Autodesk Fusion 360 part; units mm, degrees
(part 4 of 4)
  spline S181 degree 3 poles (233.08, 32.65) (233.08, 32.7604) (232.9906, 32.85) (232.88, 32.85) knots 6 6 6 6 7 7 7 7
  line L275 (233.08, 32.65) -> (233.08, 19.05)
  spline S182 degree 3 poles (232.88, 18.85) (232.9906, 18.85) (233.08, 18.9395) (233.08, 19.05) knots 4 4 4 4 5 5 5 5
  line L276 (232.88, 18.85) -> (219.2802, 18.85)
  spline S183 degree 3 poles (219.08, 19.05) (219.08, 18.9395) (219.1696, 18.85) (219.2802, 18.85) knots 2 2 2 2 3 3 3 3
  line L277 (219.08, 19.05) -> (219.08, 32.65)
  spline S184 degree 3 poles (219.2802, 32.85) (219.1696, 32.85) (219.08, 32.7604) (219.08, 32.65) knots 0 0 0 0 1 1 1 1
  line L278 (219.2802, 32.85) -> (232.88, 32.85)
  spline S185 degree 3 poles (224.0301, 51.9) (223.9197, 51.9) (223.8301, 51.8104) (223.8301, 51.7) knots 6 6 6 6 7 7 7 7
  line L279 (224.0301, 51.9) -> (237.6301, 51.9)
  spline S186 degree 3 poles (237.8301, 51.7) (237.8301, 51.8104) (237.7405, 51.9) (237.6301, 51.9) knots 4 4 4 4 5 5 5 5
  line L280 (237.8301, 51.7) -> (237.8301, 38.1)
  spline S187 degree 3 poles (237.6301, 37.9) (237.7405, 37.9) (237.8301, 37.9895) (237.8301, 38.1) knots 2 2 2 2 3 3 3 3
  line L281 (237.6301, 37.9) -> (224.0301, 37.9)
  spline S188 degree 3 poles (223.8301, 38.1) (223.8301, 37.9895) (223.9197, 37.9) (224.0301, 37.9) knots 0 0 0 0 1 1 1 1
  line L282 (223.8301, 38.1) -> (223.8301, 51.7)
  line L283 (248.0298, 7.33) -> (248.8547, 7.33)
  line L284 (248.8547, 7.33) -> (248.8547, 13.53)
  line L285 (248.8547, 13.53) -> (250.6798, 13.53)
  line L286 (250.6798, 13.53) -> (250.6798, 14.78)
  line L287 (250.6798, 14.78) -> (253.6798, 14.78)
  line L288 (253.6798, 14.78) -> (253.6798, 13.53)
  line L289 (253.6798, 13.53) -> (255.5046, 13.53)
  line L290 (255.5046, 13.53) -> (255.5046, 11.03)
  line L291 (255.5046, 11.03) -> (257.18, 11.03)
  line L292 (257.18, 11.03) -> (257.18, 13.6)
  spline S189 degree 3 poles (257.3802, 13.8) (257.2696, 13.8) (257.18, 13.7104) (257.18, 13.6) knots 28 28 28 28 29 29 29 29
  line L293 (257.3802, 13.8) -> (270.98, 13.8)
  spline S190 degree 3 poles (271.18, 13.6) (271.18, 13.7104) (271.0906, 13.8) (270.98, 13.8) knots 26 26 26 26 27 27 27 27
  line L294 (271.18, 13.6) -> (271.18, 11.03)
  line L295 (271.18, 11.03) -> (272.8557, 11.03)
  line L296 (272.8557, 11.03) -> (272.8557, 13.53)
  line L297 (272.8557, 13.53) -> (274.6807, 13.53)
  line L298 (274.6807, 13.53) -> (274.6807, 14.78)
  line L299 (274.6807, 14.78) -> (277.6807, 14.78)
  line L300 (277.6807, 14.78) -> (277.6807, 13.53)
  line L301 (277.6807, 13.53) -> (279.5058, 13.53)
  line L302 (279.5058, 13.53) -> (279.5058, 7.33)
  line L303 (279.5058, 7.33) -> (280.3307, 7.33)
  line L304 (280.3307, 7.33) -> (280.3307, 4.32)
  line L305 (280.3307, 4.32) -> (279.5058, 4.32)
  line L306 (279.5058, 4.32) -> (279.5058, 1.32)
  line L307 (279.5058, 1.32) -> (272.8557, 1.32)
  line L308 (272.8557, 1.32) -> (272.8557, 3.82)
  line L309 (272.8557, 3.82) -> (271.18, 3.82)
  line L310 (271.18, 3.82) -> (271.18, 0)
  spline S191 degree 3 poles (270.98, -0.2) (271.0906, -0.2) (271.18, -0.1105) (271.18, 0) knots 8 8 8 8 9 9 9 9
  line L311 (270.98, -0.2) -> (257.3802, -0.2)
  spline S192 degree 3 poles (257.18, 0) (257.18, -0.1105) (257.2696, -0.2) (257.3802, -0.2) knots 6 6 6 6 7 7 7 7
  line L312 (257.18, 0) -> (257.18, 3.82)
  line L313 (257.18, 3.82) -> (255.5046, 3.82)
  line L314 (255.5046, 3.82) -> (255.5046, 1.32)
  line L315 (255.5046, 1.32) -> (248.8547, 1.32)
  line L316 (248.8547, 1.32) -> (248.8547, 4.32)
  line L317 (248.8547, 4.32) -> (248.0298, 4.32)
  line L318 (248.0298, 4.32) -> (248.0298, 7.33)
  spline S193 degree 3 poles (280.5, 56.95) (280.6104, 56.95) (280.7, 57.0395) (280.7, 57.15) knots 6 6 6 6 7 7 7 7
  line L319 (280.5, 56.95) -> (266.9, 56.95)
  spline S194 degree 3 poles (266.7, 57.15) (266.7, 57.0395) (266.7896, 56.95) (266.9, 56.95) knots 4 4 4 4 5 5 5 5
  line L320 (266.7, 57.15) -> (266.7, 70.75)
  spline S195 degree 3 poles (266.9, 70.95) (266.7896, 70.95) (266.7, 70.8604) (266.7, 70.75) knots 2 2 2 2 3 3 3 3
  line L321 (266.9, 70.95) -> (280.5, 70.95)
  spline S196 degree 3 poles (280.7, 70.75) (280.7, 70.8604) (280.6104, 70.95) (280.5, 70.95) knots 0 0 0 0 1 1 1 1
  line L322 (280.7, 70.75) -> (280.7, 57.15)
  spline S197 degree 3 poles (299.55, -0.2) (299.6604, -0.2) (299.75, -0.1105) (299.75, 0) knots 6 6 6 6 7 7 7 7
  line L323 (299.55, -0.2) -> (285.95, -0.2)
  spline S198 degree 3 poles (285.75, 0) (285.75, -0.1105) (285.8396, -0.2) (285.95, -0.2) knots 4 4 4 4 5 5 5 5
  line L324 (285.75, 0) -> (285.75, 13.6)
  spline S199 degree 3 poles (285.95, 13.8) (285.8396, 13.8) (285.75, 13.7104) (285.75, 13.6) knots 2 2 2 2 3 3 3 3
  line L325 (285.95, 13.8) -> (299.55, 13.8)
  spline S200 degree 3 poles (299.75, 13.6) (299.75, 13.7104) (299.6604, 13.8) (299.55, 13.8) knots 0 0 0 0 1 1 1 1
  line L326 (299.75, 13.6) -> (299.75, 0)
  spline S201 degree 3 poles (280.5, 76) (280.6104, 76) (280.7, 76.0895) (280.7, 76.2) knots 6 6 6 6 7 7 7 7
  line L327 (280.5, 76) -> (266.9, 76)
  spline S202 degree 3 poles (266.7, 76.2) (266.7, 76.0895) (266.7896, 76) (266.9, 76) knots 4 4 4 4 5 5 5 5
  line L328 (266.7, 76.2) -> (266.7, 89.8)
  spline S203 degree 3 poles (266.9, 90) (266.7896, 90) (266.7, 89.9104) (266.7, 89.8) knots 2 2 2 2 3 3 3 3
  line L329 (266.9, 90) -> (280.5, 90)
  spline S204 degree 3 poles (280.7, 89.8) (280.7, 89.9104) (280.6104, 90) (280.5, 90) knots 0 0 0 0 1 1 1 1
  line L330 (280.7, 89.8) -> (280.7, 76.2)
  spline S205 degree 3 poles (228.1101, 56.95) (228.2205, 56.95) (228.3101, 57.0395) (228.3101, 57.15) knots 6 6 6 6 7 7 7 7
  line L331 (228.1101, 56.95) -> (214.5101, 56.95)
  spline S206 degree 3 poles (214.3101, 57.15) (214.3101, 57.0395) (214.3997, 56.95) (214.5101, 56.95) knots 4 4 4 4 5 5 5 5
  line L332 (214.3101, 57.15) -> (214.3101, 70.75)
  spline S207 degree 3 poles (214.5101, 70.95) (214.3997, 70.95) (214.3101, 70.8604) (214.3101, 70.75) knots 2 2 2 2 3 3 3 3
  line L333 (214.5101, 70.95) -> (228.1101, 70.95)
  spline S208 degree 3 poles (228.3101, 70.75) (228.3101, 70.8604) (228.2205, 70.95) (228.1101, 70.95) knots 0 0 0 0 1 1 1 1
  line L334 (228.3101, 70.75) -> (228.3101, 57.15)
  spline S209 degree 3 poles (261.45, 76) (261.5604, 76) (261.65, 76.0895) (261.65, 76.2) knots 6 6 6 6 7 7 7 7
  line L335 (261.45, 76) -> (247.85, 76)
  spline S210 degree 3 poles (247.65, 76.2) (247.65, 76.0895) (247.7396, 76) (247.85, 76) knots 4 4 4 4 5 5 5 5
  line L336 (247.65, 76.2) -> (247.65, 89.8)
  spline S211 degree 3 poles (247.85, 90) (247.7396, 90) (247.65, 89.9104) (247.65, 89.8) knots 2 2 2 2 3 3 3 3
  line L337 (247.85, 90) -> (261.45, 90)
  spline S212 degree 3 poles (261.65, 89.8) (261.65, 89.9104) (261.5604, 90) (261.45, 90) knots 0 0 0 0 1 1 1 1
  line L338 (261.65, 89.8) -> (261.65, 76.2)
  spline S213 degree 3 poles (242.4, 76) (242.5104, 76) (242.6, 76.0895) (242.6, 76.2) knots 6 6 6 6 7 7 7 7
  line L339 (242.4, 76) -> (228.8, 76)
  spline S214 degree 3 poles (228.6, 76.2) (228.6, 76.0895) (228.6896, 76) (228.8, 76) knots 4 4 4 4 5 5 5 5
  line L340 (228.6, 76.2) -> (228.6, 89.8)
  spline S215 degree 3 poles (228.8, 90) (228.6896, 90) (228.6, 89.9104) (228.6, 89.8) knots 2 2 2 2 3 3 3 3
  line L341 (228.8, 90) -> (242.4, 90)
  spline S216 degree 3 poles (242.6, 89.8) (242.6, 89.9104) (242.5104, 90) (242.4, 90) knots 0 0 0 0 1 1 1 1
  line L342 (242.6, 89.8) -> (242.6, 76.2)
  spline S217 degree 3 poles (240.705, 70.95) (240.5946, 70.95) (240.505, 70.8604) (240.505, 70.75) knots 6 6 6 6 7 7 7 7
  line L343 (240.705, 70.95) -> (254.3051, 70.95)
  spline S218 degree 3 poles (254.5051, 70.75) (254.5051, 70.8604) (254.4155, 70.95) (254.3051, 70.95) knots 4 4 4 4 5 5 5 5
  line L344 (254.5051, 70.75) -> (254.5051, 57.15)
  spline S219 degree 3 poles (254.3051, 56.95) (254.4155, 56.95) (254.5051, 57.0395) (254.5051, 57.15) knots 2 2 2 2 3 3 3 3
  line L345 (254.3051, 56.95) -> (240.705, 56.95)
  spline S220 degree 3 poles (240.505, 57.15) (240.505, 57.0395) (240.5946, 56.95) (240.705, 56.95) knots 0 0 0 0 1 1 1 1
  line L346 (240.505, 57.15) -> (240.505, 70.75)
  spline S221 degree 3 poles (157.3601, 70.95) (157.2497, 70.95) (157.1601, 70.8604) (157.1601, 70.75) knots 6 6 6 6 7 7 7 7
  line L347 (157.3601, 70.95) -> (170.9601, 70.95)
  spline S222 degree 3 poles (171.1601, 70.75) (171.1601, 70.8604) (171.0705, 70.95) (170.9601, 70.95) knots 4 4 4 4 5 5 5 5
  line L348 (171.1601, 70.75) -> (171.1601, 57.15)
  spline S223 degree 3 poles (170.9601, 56.95) (171.0705, 56.95) (171.1601, 57.0395) (171.1601, 57.15) knots 2 2 2 2 3 3 3 3
  line L349 (170.9601, 56.95) -> (157.3601, 56.95)
  spline S224 degree 3 poles (157.1601, 57.15) (157.1601, 57.0395) (157.2497, 56.95) (157.3601, 56.95) knots 0 0 0 0 1 1 1 1
  line L350 (157.1601, 57.15) -> (157.1601, 70.75)
  spline S225 degree 3 poles (180.6801, 51.7) (180.6801, 51.8104) (180.5905, 51.9) (180.4801, 51.9) knots 6 6 6 6 7 7 7 7
  line L351 (180.6801, 51.7) -> (180.6801, 38.1)
  spline S226 degree 3 poles (180.4801, 37.9) (180.5905, 37.9) (180.6801, 37.9895) (180.6801, 38.1) knots 4 4 4 4 5 5 5 5
  line L352 (180.4801, 37.9) -> (166.8801, 37.9)
  spline S227 degree 3 poles (166.6801, 38.1) (166.6801, 37.9895) (166.7697, 37.9) (166.8801, 37.9) knots 2 2 2 2 3 3 3 3
  line L353 (166.6801, 38.1) -> (166.6801, 51.7)
  spline S228 degree 3 poles (166.8801, 51.9) (166.7697, 51.9) (166.6801, 51.8104) (166.6801, 51.7) knots 0 0 0 0 1 1 1 1
  line L354 (166.8801, 51.9) -> (180.4801, 51.9)
  spline S229 degree 3 poles (152.6, 13.8) (152.4896, 13.8) (152.4, 13.7104) (152.4, 13.6) knots 6 6 6 6 7 7 7 7
  line L355 (152.6, 13.8) -> (166.2, 13.8)
  spline S230 degree 3 poles (166.4, 13.6) (166.4, 13.7104) (166.3104, 13.8) (166.2, 13.8) knots 4 4 4 4 5 5 5 5
  line L356 (166.4, 13.6) -> (166.4, 0)
  spline S231 degree 3 poles (166.2, -0.2) (166.3104, -0.2) (166.4, -0.1105) (166.4, 0) knots 2 2 2 2 3 3 3 3
  line L357 (166.2, -0.2) -> (152.6, -0.2)
  spline S232 degree 3 poles (152.4, 0) (152.4, -0.1105) (152.4896, -0.2) (152.6, -0.2) knots 0 0 0 0 1 1 1 1
  line L358 (152.4, 0) -> (152.4, 13.6)
  line L359 (143.0802, 32.85) -> (156.68, 32.85)
  spline S233 degree 3 poles (156.88, 32.65) (156.88, 32.7604) (156.7906, 32.85) (156.68, 32.85) knots 5 5 5 5 6 6 6 6
  line L360 (156.88, 32.65) -> (156.88, 19.05)
  spline S234 degree 3 poles (156.68, 18.85) (156.7906, 18.85) (156.88, 18.9395) (156.88, 19.05) knots 3 3 3 3 4 4 4 4
  line L361 (156.68, 18.85) -> (143.0802, 18.85)
  spline S235 degree 3 poles (142.88, 19.05) (142.88, 18.9395) (142.9696, 18.85) (143.0802, 18.85) knots 1 1 1 1 2 2 2 2
  line L362 (142.88, 19.05) -> (142.88, 32.65)
  spline S236 degree 3 poles (143.0802, 32.85) (142.9696, 32.85) (142.88, 32.7604) (142.88, 32.65) knots 7 7 7 7 8 8 8 8
  line L363 (104.9802, 32.85) -> (118.58, 32.85)
  spline S237 degree 3 poles (118.78, 32.65) (118.78, 32.7604) (118.6906, 32.85) (118.58, 32.85) knots 5 5 5 5 6 6 6 6
  line L364 (118.78, 32.65) -> (118.78, 19.05)
  spline S238 degree 3 poles (118.58, 18.85) (118.6906, 18.85) (118.78, 18.9395) (118.78, 19.05) knots 3 3 3 3 4 4 4 4
  line L365 (118.58, 18.85) -> (104.9802, 18.85)
  spline S239 degree 3 poles (104.78, 19.05) (104.78, 18.9395) (104.8696, 18.85) (104.9802, 18.85) knots 1 1 1 1 2 2 2 2
  line L366 (104.78, 19.05) -> (104.78, 32.65)
  spline S240 degree 3 poles (104.9802, 32.85) (104.8696, 32.85) (104.78, 32.7604) (104.78, 32.65) knots 7 7 7 7 8 8 8 8
  line L367 (162.1302, 32.85) -> (175.73, 32.85)
  spline S241 degree 3 poles (175.93, 32.65) (175.93, 32.7604) (175.8406, 32.85) (175.73, 32.85) knots 5 5 5 5 6 6 6 6
  line L368 (175.93, 32.65) -> (175.93, 19.05)
  spline S242 degree 3 poles (175.73, 18.85) (175.8406, 18.85) (175.93, 18.9395) (175.93, 19.05) knots 3 3 3 3 4 4 4 4
  line L369 (175.73, 18.85) -> (162.1302, 18.85)
  spline S243 degree 3 poles (161.93, 19.05) (161.93, 18.9395) (162.0196, 18.85) (162.1302, 18.85) knots 1 1 1 1 2 2 2 2
  line L370 (161.93, 19.05) -> (161.93, 32.65)
  spline S244 degree 3 poles (162.1302, 32.85) (162.0196, 32.85) (161.93, 32.7604) (161.93, 32.65) knots 7 7 7 7 8 8 8 8
  line L371 (85.9302, 32.85) -> (99.53, 32.85)
  spline S245 degree 3 poles (99.73, 32.65) (99.73, 32.7604) (99.6406, 32.85) (99.53, 32.85) knots 5 5 5 5 6 6 6 6
  line L372 (99.73, 32.65) -> (99.73, 19.05)
  spline S246 degree 3 poles (99.53, 18.85) (99.6406, 18.85) (99.73, 18.9395) (99.73, 19.05) knots 3 3 3 3 4 4 4 4
  line L373 (99.53, 18.85) -> (85.9302, 18.85)
  spline S247 degree 3 poles (85.73, 19.05) (85.73, 18.9395) (85.8196, 18.85) (85.9302, 18.85) knots 1 1 1 1 2 2 2 2
  line L374 (85.73, 19.05) -> (85.73, 32.65)
  spline S248 degree 3 poles (85.9302, 32.85) (85.8196, 32.85) (85.73, 32.7604) (85.73, 32.65) knots 7 7 7 7 8 8 8 8
  spline S249 degree 3 poles (138.3101, 70.95) (138.1997, 70.95) (138.1101, 70.8604) (138.1101, 70.75) knots 6 6 6 6 7 7 7 7
  line L375 (138.3101, 70.95) -> (151.9101, 70.95)
  spline S250 degree 3 poles (152.1101, 70.75) (152.1101, 70.8604) (152.0205, 70.95) (151.9101, 70.95) knots 4 4 4 4 5 5 5 5
  line L376 (152.1101, 70.75) -> (152.1101, 57.15)
  spline S251 degree 3 poles (151.9101, 56.95) (152.0205, 56.95) (152.1101, 57.0395) (152.1101, 57.15) knots 2 2 2 2 3 3 3 3
  line L377 (151.9101, 56.95) -> (138.3101, 56.95)
  spline S252 degree 3 poles (138.1101, 57.15) (138.1101, 57.0395) (138.1997, 56.95) (138.3101, 56.95) knots 0 0 0 0 1 1 1 1
  line L378 (138.1101, 57.15) -> (138.1101, 70.75)
  spline S253 degree 3 poles (52.5801, 51.9) (52.4697, 51.9) (52.3801, 51.8104) (52.3801, 51.7) knots 6 6 6 6 7 7 7 7
  line L379 (52.5801, 51.9) -> (66.1801, 51.9)
  spline S254 degree 3 poles (66.3801, 51.7) (66.3801, 51.8104) (66.2905, 51.9) (66.1801, 51.9) knots 4 4 4 4 5 5 5 5
  line L380 (66.3801, 51.7) -> (66.3801, 38.1)
  spline S255 degree 3 poles (66.1801, 37.9) (66.2905, 37.9) (66.3801, 37.9895) (66.3801, 38.1) knots 2 2 2 2 3 3 3 3
  line L381 (66.1801, 37.9) -> (52.5801, 37.9)
  spline S256 degree 3 poles (52.3801, 38.1) (52.3801, 37.9895) (52.4697, 37.9) (52.5801, 37.9) knots 0 0 0 0 1 1 1 1
  line L382 (52.3801, 38.1) -> (52.3801, 51.7)
  line L383 (66.8802, 32.85) -> (80.48, 32.85)
  spline S257 degree 3 poles (80.68, 32.65) (80.68, 32.7604) (80.5906, 32.85) (80.48, 32.85) knots 5 5 5 5 6 6 6 6
  line L384 (80.68, 32.65) -> (80.68, 19.05)
  spline S258 degree 3 poles (80.48, 18.85) (80.5906, 18.85) (80.68, 18.9395) (80.68, 19.05) knots 3 3 3 3 4 4 4 4
  line L385 (80.48, 18.85) -> (66.8802, 18.85)
  spline S259 degree 3 poles (66.68, 19.05) (66.68, 18.9395) (66.7696, 18.85) (66.8802, 18.85) knots 1 1 1 1 2 2 2 2
  line L386 (66.68, 19.05) -> (66.68, 32.65)
  spline S260 degree 3 poles (66.8802, 32.85) (66.7696, 32.85) (66.68, 32.7604) (66.68, 32.65) knots 7 7 7 7 8 8 8 8
  spline S261 degree 3 poles (114.5, 13.8) (114.3896, 13.8) (114.3, 13.7104) (114.3, 13.6) knots 6 6 6 6 7 7 7 7
  line L387 (114.5, 13.8) -> (128.1, 13.8)
  spline S262 degree 3 poles (128.3, 13.6) (128.3, 13.7104) (128.2104, 13.8) (128.1, 13.8) knots 4 4 4 4 5 5 5 5
  line L388 (128.3, 13.6) -> (128.3, 0)
  spline S263 degree 3 poles (128.1, -0.2) (128.2104, -0.2) (128.3, -0.1105) (128.3, 0) knots 2 2 2 2 3 3 3 3
  line L389 (128.1, -0.2) -> (114.5, -0.2)
  spline S264 degree 3 poles (114.3, 0) (114.3, -0.1105) (114.3896, -0.2) (114.5, -0.2) knots 0 0 0 0 1 1 1 1
  line L390 (114.3, 0) -> (114.3, 13.6)
  spline S265 degree 3 poles (214.03, 32.65) (214.03, 32.7604) (213.9406, 32.85) (213.83, 32.85) knots 6 6 6 6 7 7 7 7
  line L391 (214.03, 32.65) -> (214.03, 19.05)
  spline S266 degree 3 poles (213.83, 18.85) (213.9406, 18.85) (214.03, 18.9395) (214.03, 19.05) knots 4 4 4 4 5 5 5 5
  line L392 (213.83, 18.85) -> (200.2302, 18.85)
  spline S267 degree 3 poles (200.03, 19.05) (200.03, 18.9395) (200.1196, 18.85) (200.2302, 18.85) knots 2 2 2 2 3 3 3 3
  line L393 (200.03, 19.05) -> (200.03, 32.65)
  spline S268 degree 3 poles (200.2302, 32.85) (200.1196, 32.85) (200.03, 32.7604) (200.03, 32.65) knots 0 0 0 0 1 1 1 1
  line L394 (200.2302, 32.85) -> (213.83, 32.85)
  spline S269 degree 3 poles (171.65, 13.8) (171.5396, 13.8) (171.45, 13.7104) (171.45, 13.6) knots 6 6 6 6 7 7 7 7
  line L395 (171.65, 13.8) -> (185.25, 13.8)
  spline S270 degree 3 poles (185.45, 13.6) (185.45, 13.7104) (185.3604, 13.8) (185.25, 13.8) knots 4 4 4 4 5 5 5 5
  line L396 (185.45, 13.6) -> (185.45, 0)
  spline S271 degree 3 poles (185.25, -0.2) (185.3604, -0.2) (185.45, -0.1105) (185.45, 0) knots 2 2 2 2 3 3 3 3
  line L397 (185.25, -0.2) -> (171.65, -0.2)
  spline S272 degree 3 poles (171.45, 0) (171.45, -0.1105) (171.5396, -0.2) (171.65, -0.2) knots 0 0 0 0 1 1 1 1
  line L398 (171.45, 0) -> (171.45, 13.6)
  arc A8 (-5, 103) -> (-13, 95) centre (-5, 95) ccw
  line L399 (-13, 95) -> (-13, -5.2)
  arc A9 (-13, -5.2) -> (-5, -13.2) centre (-5, -5.2) ccw
  line L400 (-5, -13.2) -> (304.75, -13.2)
  arc A10 (304.75, -13.2) -> (312.75, -5.2) centre (304.75, -5.2) ccw
  line L401 (312.75, -5.2) -> (312.75, 95)
  arc A11 (312.75, 95) -> (304.75, 103) centre (304.75, 95) ccw
  line L402 (304.75, 103) -> (-5, 103)
  circle A12 centre (307.75, -8.2) radius 1.5
  circle A13 centre (228.8125, -8.2) radius 1.5
  circle A14 centre (70.9375, -8.2) radius 1.5
  circle A15 centre (-8, -8.2) radius 1.5
  circle A16 centre (-8, 98) radius 1.5
  circle A17 centre (70.9375, 98) radius 1.5
  circle A18 centre (228.8125, 98) radius 1.5
  circle A19 centre (307.75, 98) radius 1.5
  line L403 (302.75, -3.2) -> (-3, -3.2)
  line L404 (-3, -3.2) -> (-3, 93)
  line L405 (-3, 93) -> (302.75, 93)
  line L406 (302.75, 93) -> (302.75, -3.2)
  line L407 (-13, 11.8) -> (-3, 11.8)
  line L408 (-3, 71.8) -> (-13, 71.8)
  line L409 (-13, 11.8) -> (-13, -5.2)
  line L410 (-13, 71.8) -> (-13, 95)
  dimension "d343" = 3
  dimension "d363" = 3
  dimension "d364" = 3
  dimension "d365" = 3
  dimension "d410" = 60
  dimension "d411" = 15
  constraint concentric A1 A12
  constraint concentric A0 A13
  constraint concentric A5 A14
  constraint concentric A4 A15
  constraint concentric A3 A16
  constraint concentric A6 A17
  constraint concentric A7 A18
  constraint concentric A2 A19
  constraint equal A13 A14
  constraint equal A14 A15
  constraint equal A15 A16
  constraint equal A16 A17
  constraint equal A17 A18
  constraint equal A18 A19
  constraint equal A12 A13
  constraint horizontal L403
  constraint vertical L404
  constraint horizontal L405
  constraint vertical L406
  constraint coincident L399 L407.start
  constraint coincident L404 L407.end
  constraint perpendicular L404 L407
  constraint coincident L404 L408.start
  constraint coincident L399 L408.end
  constraint perpendicular L399 L408
  constraint coincident L399.end A9.start
  constraint coincident A8.end L399.start
  measures "d343" diameter of A12
  measures "d363" distance of L35 L404
  measures "d364" distance of L34 L403
  measures "d365" distance of L257 L405
  measures "d410" distance of L407 L408
  measures "d411" distance of L403 L407
extrude "Extrude5" add sketch "Sketch1" along normal blind 3 separate body contours A8 L399 A9 L400 A10 L401 A11 L402 L403 L404 L405 L406 L407 L408 L409 L410 makes body 4 in component "usb-plate"
sketch "Sketch1 (2)" plane through (0, 0, -9) normal (0, 0, -1) x (1, 0, 0) in component "battery-plate"
  circle A0 centre (307.75, 98) radius 1.5
  circle A1 centre (228.8125, 98) radius 1.5
  circle A2 centre (70.9375, 98) radius 1.5
  circle A3 centre (70.9375, -8.2) radius 1.5
  circle A4 centre (228.8125, -8.2) radius 1.5
  circle A5 centre (-8, 98) radius 1.5
  circle A6 centre (-8, -8.2) radius 1.5
  circle A7 centre (307.75, -8.2) radius 1.5
  line L0 (302.75, 93) -> (302.75, -3.2)
  line L1 (312.75, -5.2) -> (312.75, 95)
  arc A8 (312.75, 95) -> (304.75, 103) centre (304.75, 95) ccw
  line L2 (304.75, 103) -> (-5, 103)
  arc A9 (-5, 103) -> (-13, 95) centre (-5, 95) ccw
  line L3 (-13, 95) -> (-13, -5.2)
  arc A10 (-13, -5.2) -> (-5, -13.2) centre (-5, -5.2) ccw
  line L4 (-5, -13.2) -> (304.75, -13.2)
  arc A11 (304.75, -13.2) -> (312.75, -5.2) centre (304.75, -5.2) ccw
  line L5 (302.75, -3.2) -> (-3, -3.2)
  line L6 (-3, -3.2) -> (-3, 93)
  line L7 (-3, 93) -> (302.75, 93)
  line L8 (302.75, -3.2) -> (-3, -3.2)
  line L9 (-3, -3.2) -> (-3, 93)
  line L10 (-3, 93) -> (302.75, 93)
  line L11 (302.75, 93) -> (302.75, -3.2)
  line L12 (312.75, 14.8) -> (302.75, 14.8)
  line L13 (302.75, 14.8) -> (302.75, -3.2)
  line L14 (302.75, -3.2) -> (312.75, -3.2)
  line L15 (312.75, -3.2) -> (312.75, 14.8)
  line L16 (149.875, -13.2) -> (149.875, 103) construction
  line L17 (-13, 44.9) -> (312.75, 44.9) construction
  line L18 (199.875, 9.9) -> (99.875, 9.9)
  line L19 (99.875, 9.9) -> (99.875, 79.9)
  line L20 (99.875, 79.9) -> (199.875, 79.9)
  line L21 (199.875, 79.9) -> (199.875, 9.9)
  circle A12 centre (228.8125, -8.2) radius 1.5
  circle A13 centre (70.9375, -8.2) radius 1.5
  circle A14 centre (-8, -8.2) radius 1.5
  circle A15 centre (-8, 98) radius 1.5
  circle A16 centre (70.9375, 98) radius 1.5
  circle A17 centre (228.8125, 98) radius 1.5
  circle A18 centre (307.75, 98) radius 1.5
  circle A19 centre (307.75, -8.2) radius 1.5
  line L22 (-3, 71.8) -> (-3, 93)
  line L23 (-3, 93) -> (302.75, 93)
  line L24 (302.75, 93) -> (302.75, -3.2)
  line L25 (302.75, -3.2) -> (-3, -3.2)
  line L26 (-3, -3.2) -> (-3, 11.8)
  line L27 (-3, 11.8) -> (-13, 11.8)
  line L28 (-13, 11.8) -> (-13, -5.2)
  arc A20 (-13, -5.2) -> (-5, -13.2) centre (-5, -5.2) ccw
  line L29 (-5, -13.2) -> (304.75, -13.2)
  arc A21 (304.75, -13.2) -> (312.75, -5.2) centre (304.75, -5.2) ccw
  line L30 (312.75, -5.2) -> (312.75, 95)
  arc A22 (312.75, 95) -> (304.75, 103) centre (304.75, 95) ccw
  line L31 (304.75, 103) -> (-5, 103)
  arc A23 (-5, 103) -> (-13, 95) centre (-5, 95) ccw
  line L32 (-13, 95) -> (-13, 71.8)
  line L33 (-13, 71.8) -> (-3, 71.8)
  dimension "d377" = 100
  dimension "d378" = 70
  constraint horizontal L8
  constraint vertical L9
  constraint horizontal L10
  constraint vertical L11
  constraint coincident L6.end L7.start
  constraint coincident L0.end L5.start
  constraint horizontal L12
  constraint vertical L13
  constraint horizontal L14
  constraint vertical L15
  constraint midpoint L4 L16.start
  constraint midpoint L2 L16.end
  constraint midpoint L3 L17.start
  constraint coincident L15 L17.end
  constraint perpendicular L15 L17
  constraint horizontal L18
  constraint vertical L19
  constraint horizontal L20
  constraint vertical L21
  constraint symmetric L16 L18.start L18.end
  constraint symmetric L17 L18.end L19.end
  measures "d377" distance of L19 L21
  measures "d378" distance of L18 L20
extrude "Extrude1'" add sketch "Sketch1 (2)" along normal blind 3 separate body makes body 5 in component "battery-plate"
sketch "Sketch1 (3)" plane through (0, 0, -12) normal (0, 0, -1) x (1, 0, 0) in component "bottom-plate"
  arc A0 (312.75, 95) -> (304.75, 103) centre (304.75, 95) ccw
  line L0 (304.75, 103) -> (-5, 103)
  arc A1 (-5, 103) -> (-13, 95) centre (-5, 95) ccw
  line L1 (-13, 95) -> (-13, -5.2)
  arc A2 (-13, -5.2) -> (-5, -13.2) centre (-5, -5.2) ccw
  line L2 (-5, -13.2) -> (304.75, -13.2)
  arc A3 (304.75, -13.2) -> (312.75, -5.2) centre (304.75, -5.2) ccw
  line L3 (312.75, -5.2) -> (312.75, 95)
  line L4 (287.75, -0.1) -> (284.75, -0.1)
  line L5 (284.75, -0.1) -> (284.75, 89.9)
  line L6 (284.75, 89.9) -> (287.75, 89.9)
  line L7 (287.75, 89.9) -> (287.75, -0.1)
  line L8 (281.75, -0.1) -> (278.75, -0.1)
  line L9 (278.75, -0.1) -> (278.75, 89.9)
  line L10 (278.75, 89.9) -> (281.75, 89.9)
  line L11 (281.75, 89.9) -> (281.75, -0.1)
  line L12 (312.75, 44.9) -> (-13, 44.9) construction
  line L13 (149.875, -13.2) -> (149.875, 103) construction
  line L14 (15, -0.1) -> (12, -0.1)
  line L15 (18, -0.1) -> (18, 89.9)
  line L16 (21, -0.1) -> (18, -0.1)
  line L17 (62.75, 44.9) -> (-263, 44.9) construction
  line L18 (21, 89.9) -> (21, -0.1)
  line L19 (15, 89.9) -> (15, -0.1)
  line L20 (12, 89.9) -> (15, 89.9)
  line L21 (12, -0.1) -> (12, 89.9)
  line L22 (18, 89.9) -> (21, 89.9)
  line L23 (12, 21.6249) -> (-13, 21.6249) construction
  line L24 (312.75, 18.2437) -> (287.75, 18.2437) construction
  circle A4 centre (307.75, -8.2) radius 1
  circle A5 centre (228.8125, -8.2) radius 1
  circle A6 centre (70.9375, -8.2) radius 1
  circle A7 centre (-8, -8.2) radius 1
  circle A8 centre (-8, 98) radius 1
  circle A9 centre (70.9375, 98) radius 1
  circle A10 centre (228.8125, 98) radius 1
  circle A11 centre (307.75, 98) radius 1
  dimension "d381" = 3
  dimension "d382" = 90
  dimension "d383" = 3
  dimension "d386" = 3
  dimension "d387" = 25
  dimension "d400" = 2
  constraint horizontal L4
  constraint vertical L5
  constraint horizontal L6
  constraint vertical L7
  constraint horizontal L8
  constraint vertical L9
  constraint horizontal L10
  constraint vertical L11
  constraint collinear L4 L8
  constraint collinear L6 L10
  constraint equal L6 L10
  constraint midpoint L3 L12.start
  constraint midpoint L1 L12.end
  constraint midpoint L2 L13.start
  constraint midpoint L0 L13.end
  constraint symmetric L4.start L6.end L12
  constraint horizontal L16
  constraint vertical L15
  constraint horizontal L22
  constraint vertical L18
  constraint horizontal L14
  constraint vertical L21
  constraint horizontal L20
  constraint vertical L19
  constraint collinear L14 L16
  constraint collinear L20 L22
  constraint equal L20 L22
  constraint symmetric L18.start L16.start L17
  constraint equal L4 L16
  constraint coincident L21 L23.start
  constraint coincident L1 L23.end
  constraint perpendicular L1 L23
  constraint coincident L3 L24.start
  constraint coincident L7 L24.end
  constraint perpendicular L7 L24
  constraint equal L23 L24
  constraint equal A4 A5
  constraint equal A5 A6
  constraint equal A6 A7
  constraint equal A7 A8
  constraint equal A8 A9
  constraint equal A10 A11
  constraint equal A9 A10
  measures "d381" distance of L4.start L4.end
  measures "d382" distance of L4 L6
  measures "d383" distance of L5 L11
  measures "d386" distance of L15 L19
  measures "d387" distance of L3 L7
  measures "d400" diameter of A4
extrude "Extrude2''" add sketch "Sketch1 (3)" along normal blind 3 separate body makes body 6 in component "bottom-plate"
sketch "Sketch1 (4)" plane through (12, 0, 0) normal (1, 0, 0) x (0, 1, 0) in component "feet_01"
  line L0 (0.1, -12) -> (-89.9, -12)
  line L1 (-89.9, -12) -> (-89.9, -15)
  line L2 (-89.9, -15) -> (0.1, -15)
  line L3 (0.1, -15) -> (0.1, -12)
  line L4 (0.1, -15) -> (0.1, -18.6714)
  line L5 (-3.0399, -21.6682) -> (-87.0399, -17.7472)
  line L6 (-89.9, -15) -> (-89.9, -14.7504)
  line L7 (-89.9, -17.6137) -> (-102.9755, -17.0033) construction
  line L8 (-103, -15) -> (-103.0933, -16.9978) construction
  arc A0 (-3.0399, -21.6682) -> (0.1, -18.6714) centre (-2.9, -18.6714) ccw
  arc A1 (-89.9, -14.7504) -> (-87.0399, -17.7472) centre (-86.9, -14.7504) ccw
  line L9 (-2.9, -18.6714) -> (-21.4301, -17.8065) construction
  circle A2 centre (-21.4301, -17.8065) radius 1
  circle A3 centre (-2.9, -18.6714) radius 1
  line L10 (0.1, -12) -> (-89.9, -12)
  line L11 (-89.9, -12) -> (-89.9, -15)
  line L12 (-89.9, -15) -> (0.1, -15)
  line L13 (0.1, -15) -> (0.1, -12)
  point P0 (-103, -15)
  dimension "d390" = 2
  dimension "d392" = 3
  dimension "d393" = 2
  constraint coincident L2.end L3.start
  constraint perpendicular L2 L4
  constraint coincident L1.end L2.start
  constraint vertical L6
  constraint parallel L5 L7
  constraint coincident L7 L8.end
  constraint perpendicular L7 L8
  constraint tangent L5 A0
  constraint tangent L4 A0
  constraint coincident L7.start L6
  constraint coincident L7.start L5
  constraint tangent L6 A1
  constraint tangent L5 A1
  constraint coincident A0.centre L9.start
  constraint coincident P0 L8.start
  constraint coincident L9.end A2.centre
  constraint concentric A0 A3
  constraint equal A2 A3
  constraint parallel L5 L9
  constraint equal A0 A1
  measures "d390" distance of P0 L8.end
  measures "d392" radius of A1
  measures "d393" diameter of A2
extrude "Extrude1''" add sketch "Sketch1 (4)" along normal blind 3 separate body contours L0 L1 L2 L3 A1 L10 L11 L12 L13 | L2 L4 L5 A0 A1 L12 makes body 7 in component "feet_01"
sketch "Sketch1 (5)" plane through (15, 0, 0) normal (1, 0, 0) x (0, 1, 0) in component "feet_02"
  circle A0 centre (-21.4301, -17.8065) radius 1
  circle A1 centre (-2.9, -18.6714) radius 1
  line L0 (0.1, -18.6714) -> (0.1, -12)
  line L1 (0.1, -12) -> (-89.9, -12)
  line L2 (-89.9, -12) -> (-89.9, -14.7504)
  arc A2 (-89.9, -14.7504) -> (-87.0399, -17.7472) centre (-86.9, -14.7504) ccw
  line L3 (-87.0399, -17.7472) -> (-3.0399, -21.6682)
  arc A3 (-3.0399, -21.6682) -> (0.1, -18.6714) centre (-2.9, -18.6714) ccw
  line L4 (-89.9, -14.9938) -> (0.1, -14.9938)
  constraint coincident L2 L4.start
  constraint coincident L0 L4.end
  constraint perpendicular L0 L4
extrude "Extrude1'''" add sketch "Sketch1 (5)" along normal blind 3 separate body contours L0 A2 L3 A3 L4 makes body 8 in component "feet_02"
sketch "Sketch2" plane through (0, 0, 7.5) normal (0, 0, 1) x (-1, 0, 0) in component "top-plate"
  circle A0 centre (8, -8.2) radius 1
  circle A1 centre (-70.9375, -8.2) radius 1
  line L0 (3, -3.2) -> (-302.75, -3.2)
  line L1 (-302.75, -3.2) -> (-302.75, 93)
  line L2 (-302.75, 93) -> (3, 93)
  line L3 (3, 93) -> (3, -3.2)
  circle A2 centre (-228.8125, 98) radius 1
  circle A3 centre (-70.9375, 98) radius 1
  circle A4 centre (-228.8125, -8.2) radius 1
  circle A5 centre (-307.75, -8.2) radius 1
  circle A6 centre (-307.75, 98) radius 1
  circle A7 centre (8, 98) radius 1
  arc A8 (-310.25, 7.758) -> (-312.75, 4.8) centre (-309.75, 4.8) ccw
  line L4 (-312.75, 4.8) -> (-312.75, -5.2)
  arc A9 (-312.75, -5.2) -> (-304.75, -13.2) centre (-304.75, -5.2) ccw
  line L5 (-304.75, -13.2) -> (5, -13.2)
  arc A10 (5, -13.2) -> (13, -5.2) centre (5, -5.2) ccw
  line L6 (13, -5.2) -> (13, 4.8)
  arc A11 (13, 4.8) -> (10.5, 7.758) centre (10, 4.8) ccw
  arc A12 (8, 10.7161) -> (10.5, 7.758) centre (11, 10.7161) ccw
  line L7 (8, 10.7161) -> (8, 79.0839)
  arc A13 (10.5, 82.042) -> (8, 79.0839) centre (11, 79.0839) ccw
  arc A14 (10.5, 82.042) -> (13, 85) centre (10, 85) ccw
  line L8 (13, 85) -> (13, 95)
  arc A15 (13, 95) -> (5, 103) centre (5, 95) ccw
  line L9 (5, 103) -> (-304.75, 103)
  arc A16 (-304.75, 103) -> (-312.75, 95) centre (-304.75, 95) ccw
  line L10 (-312.75, 95) -> (-312.75, 85)
  arc A17 (-312.75, 85) -> (-310.25, 82.042) centre (-309.75, 85) ccw
  arc A18 (-307.75, 79.0839) -> (-310.25, 82.042) centre (-310.75, 79.0839) ccw
  line L11 (-307.75, 79.0839) -> (-307.75, 10.7161)
  arc A19 (-310.25, 7.758) -> (-307.75, 10.7161) centre (-310.75, 10.7161) ccw
sketch "Sketch2 (2)" plane through (0, 0, 4.5) normal (0, 0, 1) x (-1, 0, 0) in component "led-plate"
  circle A0 centre (-307.75, 98) radius 1
  circle A1 centre (8, 98) radius 1
  circle A2 centre (-307.75, -8.2) radius 1
  circle A3 centre (-228.8125, -8.2) radius 1
  line L0 (-302.75, 93) -> (3, 93)
  line L1 (3, 93) -> (3, -3.2)
  line L2 (3, -3.2) -> (-302.75, -3.2)
  line L3 (-302.75, -3.2) -> (-302.75, 93)
  circle A4 centre (-228.8125, 98) radius 1
  circle A5 centre (-70.9375, 98) radius 1
  circle A6 centre (-70.9375, -8.2) radius 1
  circle A7 centre (8, -8.2) radius 1
  line L4 (13, -5.2) -> (13, 95)
  arc A8 (13, 95) -> (5, 103) centre (5, 95) ccw
  line L5 (5, 103) -> (-304.75, 103)
  arc A9 (-304.75, 103) -> (-312.75, 95) centre (-304.75, 95) ccw
  line L6 (-312.75, 95) -> (-312.75, -5.2)
  arc A10 (-312.75, -5.2) -> (-304.75, -13.2) centre (-304.75, -5.2) ccw
  line L7 (-304.75, -13.2) -> (5, -13.2)
  arc A11 (5, -13.2) -> (13, -5.2) centre (5, -5.2) ccw
sketch "Sketch3" plane through (0, 0, 0) normal (0, 0, 1) x (-1, 0, 0) in component "usb-plate"
  circle A0 centre (-228.8125, -8.2) radius 1.5
  circle A1 centre (-70.9375, -8.2) radius 1.5
  circle A2 centre (8, -8.2) radius 1.5
  circle A3 centre (8, 98) radius 1.5
  circle A4 centre (-70.9375, 98) radius 1.5
  circle A5 centre (-228.8125, 98) radius 1.5
  circle A6 centre (-307.75, 98) radius 1.5
  circle A7 centre (-307.75, -8.2) radius 1.5
  line L0 (3, 93) -> (3, 71.8)
  line L1 (3, 71.8) -> (13, 71.8)
  line L2 (13, 71.8) -> (13, 95)
  arc A8 (13, 95) -> (5, 103) centre (5, 95) ccw
  line L3 (5, 103) -> (-304.75, 103)
  arc A9 (-304.75, 103) -> (-312.75, 95) centre (-304.75, 95) ccw
  line L4 (-312.75, 95) -> (-312.75, -5.2)
  arc A10 (-312.75, -5.2) -> (-304.75, -13.2) centre (-304.75, -5.2) ccw
  line L5 (-304.75, -13.2) -> (5, -13.2)
  arc A11 (5, -13.2) -> (13, -5.2) centre (5, -5.2) ccw
  line L6 (13, -5.2) -> (13, 11.8)
  line L7 (13, 11.8) -> (3, 11.8)
  line L8 (3, 11.8) -> (3, -3.2)
  line L9 (3, -3.2) -> (-302.75, -3.2)
  line L10 (-302.75, -3.2) -> (-302.75, 93)
  line L11 (-302.75, 93) -> (3, 93)
sketch "Sketch3 (2)" plane through (0, 0, -9) normal (0, 0, 1) x (-1, 0, 0) in component "battery-plate"
  circle A0 centre (-307.75, 98) radius 1.5
  line L0 (-199.875, 79.9) -> (-99.875, 79.9)
  line L1 (-99.875, 79.9) -> (-99.875, 9.9)
  line L2 (-99.875, 9.9) -> (-199.875, 9.9)
  line L3 (-199.875, 9.9) -> (-199.875, 79.9)
  circle A1 centre (-70.9375, -8.2) radius 1.5
  circle A2 centre (-228.8125, 98) radius 1.5
  circle A3 centre (-70.9375, 98) radius 1.5
  circle A4 centre (8, 98) radius 1.5
  circle A5 centre (8, -8.2) radius 1.5
  circle A6 centre (-307.75, -8.2) radius 1.5
  circle A7 centre (-228.8125, -8.2) radius 1.5
  line L4 (-312.75, 95) -> (-312.75, -5.2)
  arc A8 (-312.75, -5.2) -> (-304.75, -13.2) centre (-304.75, -5.2) ccw
  line L5 (-304.75, -13.2) -> (5, -13.2)
  arc A9 (5, -13.2) -> (13, -5.2) centre (5, -5.2) ccw
  line L6 (13, -5.2) -> (13, 95)
  arc A10 (13, 95) -> (5, 103) centre (5, 95) ccw
  line L7 (5, 103) -> (-304.75, 103)
  arc A11 (-304.75, 103) -> (-312.75, 95) centre (-304.75, 95) ccw
sketch "Sketch2 (3)" plane through (0, 0, -12) normal (0, 0, 1) x (-1, 0, 0) in component "bottom-plate"
  line L0 (-12, -0.1) -> (-15, -0.1)
  line L1 (-15, -0.1) -> (-15, 89.9)
  line L2 (-15, 89.9) -> (-12, 89.9)
  line L3 (-12, 89.9) -> (-12, -0.1)
  circle A0 centre (-228.8125, -8.2) radius 1
  line L4 (-18, 89.9) -> (-18, -0.1)
  line L5 (-18, -0.1) -> (-21, -0.1)
  line L6 (-21, -0.1) -> (-21, 89.9)
  line L7 (-21, 89.9) -> (-18, 89.9)
  circle A1 centre (-70.9375, -8.2) radius 1
  circle A2 centre (-307.75, -8.2) radius 1
  circle A3 centre (8, -8.2) radius 1
  circle A4 centre (8, 98) radius 1
  circle A5 centre (-70.9375, 98) radius 1
  circle A6 centre (-228.8125, 98) radius 1
  circle A7 centre (-307.75, 98) radius 1
  line L8 (-281.75, 89.9) -> (-278.75, 89.9)
  line L9 (-278.75, 89.9) -> (-278.75, -0.1)
  line L10 (-278.75, -0.1) -> (-281.75, -0.1)
  line L11 (-281.75, -0.1) -> (-281.75, 89.9)
  line L12 (-287.75, 89.9) -> (-284.75, 89.9)
  line L13 (-284.75, 89.9) -> (-284.75, -0.1)
  line L14 (-284.75, -0.1) -> (-287.75, -0.1)
  line L15 (-287.75, -0.1) -> (-287.75, 89.9)
  line L16 (-312.75, 95) -> (-312.75, -5.2)
  arc A8 (-312.75, -5.2) -> (-304.75, -13.2) centre (-304.75, -5.2) ccw
  line L17 (-304.75, -13.2) -> (5, -13.2)
  arc A9 (5, -13.2) -> (13, -5.2) centre (5, -5.2) ccw
  line L18 (13, -5.2) -> (13, 95)
  arc A10 (13, 95) -> (5, 103) centre (5, 95) ccw
  line L19 (5, 103) -> (-304.75, 103)
  arc A11 (-304.75, 103) -> (-312.75, 95) centre (-304.75, 95) ccw
sketch "Sketch2 (4)" plane through (12, 0, 0) normal (-1, 0, 0) x (0, -1, 0) in component "feet_01"
  circle A0 centre (21.4301, -17.8065) radius 1
  circle A1 centre (2.9, -18.6714) radius 1
  line L0 (-0.1, -12) -> (-0.1, -18.6714)
  arc A2 (-0.1, -18.6714) -> (3.0399, -21.6682) centre (2.9, -18.6714) ccw
  line L1 (3.0399, -21.6682) -> (87.0399, -17.7472)
  arc A3 (87.0399, -17.7472) -> (89.9, -14.7504) centre (86.9, -14.7504) ccw
  line L2 (89.9, -14.7504) -> (89.9, -12)
  line L3 (89.9, -12) -> (-0.1, -12)
sketch "Sketch2 (5)" plane through (15, 0, 0) normal (-1, 0, 0) x (0, -1, 0) in component "feet_02"
  circle A0 centre (21.4301, -17.8065) radius 1
  circle A1 centre (2.9, -18.6714) radius 1
  line L0 (3.0399, -21.6682) -> (87.0399, -17.7472)
  arc A2 (87.0399, -17.7472) -> (89.8901, -14.9938) centre (86.9, -14.7504) ccw
  line L1 (89.8901, -14.9938) -> (-0.1, -14.9938)
  line L2 (-0.1, -14.9938) -> (-0.1, -18.6714)
  arc A3 (-0.1, -18.6714) -> (3.0399, -21.6682) centre (2.9, -18.6714) ccw
component "switch-plate" placed x (1, 0, 0) y (0, 1, 0) z (0, 0, 1) at (0, 0, 0)
component "led-plate" placed x (1, 0, 0) y (0, 1, 0) z (0, 0, 1) at (0, 0, 0)
component "top-plate" placed x (1, 0, 0) y (0, 1, 0) z (0, 0, 1) at (0, 0, 0)
component "usb-plate" placed x (1, 0, 0) y (0, 1, 0) z (0, 0, 1) at (0, 0, 0)
component "usb-plate" placed x (1, 0, 0) y (0, 1, 0) z (0, 0, 1) at (0, 0, -3)
component "usb-plate" placed x (1, 0, 0) y (0, 1, 0) z (0, 0, 1) at (0, 0, -6)
component "battery-plate" placed x (1, 0, 0) y (0, 1, 0) z (0, 0, 1) at (0, 0, 0)
component "bottom-plate" placed x (1, 0, 0) y (0, 1, 0) z (0, 0, 1) at (0, 0, 0)
component "feet_01" placed x (1, 0, 0) y (0, 1, 0) z (0, 0, 1) at (0, 0, 0)
component "feet_02" placed x (1, 0, 0) y (0, 1, 0) z (0, 0, 1) at (0, 0, 0)
component "feet_01" placed x (1, 0, 0) y (0, 1, 0) z (0, 0, 1) at (6, 0, 0)
equation "cornerRadius = 8 mm"
equation "bezelWidth = 10 mm"
equation "holeDiameter01 = 2 mm"
equation "keycapDistance = 3 mm"
equation "switchHole = 14 mm"
equation "batteryWidth = 100 mm"
equation "batteryHeight = 70 mm"
equation "holeDiameter02 = 3 mm"
equation "d289 = bezelWidth / 2"
equation "d290 = bezelWidth"
equation "d291 = bezelWidth / 2"
equation "d292 = bezelWidth"
equation "d294 = bezelWidth / 2"
equation "d295 = bezelWidth"
equation "d301 = bezelWidth / 2"
equation "d302 = bezelWidth"
equation "d303 = cornerRadius"
equation "d377 = batteryWidth"
equation "d378 = batteryHeight"
equation "d390 = holeDiameter01"
equation "d393 = holeDiameter01"
equation "usbLength = 50 mm"
